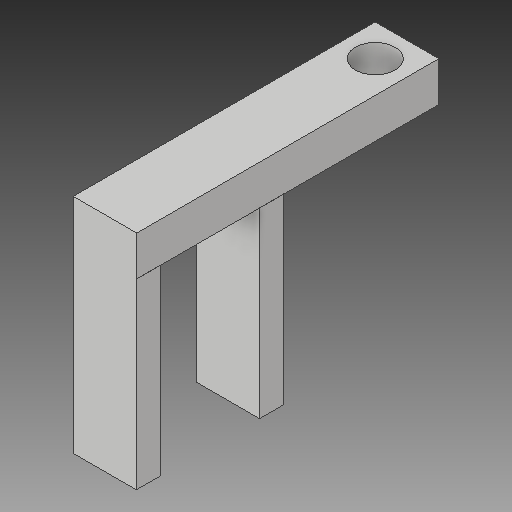
# Autodesk Inventor part: A1
Saved by Autodesk Inventor 2019 (Build 230136000, 136)
## iProperties
Created: 2020-03-28
Part Number: A1
Material: Generic
Document SubType Name: Modeling
Designer: Pulag
Density: 1 g/cm^3
Appearance: Default
Author: Pulag
Autodesk Inventor part; units mm, degrees
ref_plane "YZ Plane" through (0, 0, 0) normal (1, 0, 0) x (0, 1, 0)
ref_plane "XZ Plane" through (0, 0, 0) normal (0, 1, 0) x (-1, 0, 0)
ref_plane "XY Plane" through (0, 0, 0) normal (0, 0, 1) x (1, 0, 0)
sketch "Sketch1" plane through (0, 0, 0) normal (0, 1, 0) x (-1, 0, 0)
  point P0 (0, 0)
sketch "Sketch2" plane through (-2.6971, 0, -13.0721) normal (0, 1, 0) x (-1, 0, 0)
  circle A0 centre (-1.6971, 1.6971) radius 2.5
  line L0 (2.3029, 5.6971) -> (-5.6971, 5.6971)
  line L1 (-5.6971, 5.6971) -> (-5.6971, -2.3029)
  line L2 (-5.6971, -2.3029) -> (2.3029, -2.3029)
  line L3 (2.3029, -2.3029) -> (2.3029, 5.6971)
  line L4 (2.3029, 5.6971) -> (-5.6971, -2.3029) construction
  line L5 (-5.6971, 5.6971) -> (2.3029, -2.3029) construction
  line L6 (2.3029, 5.6971) -> (-5.6971, 5.6971)
  line L7 (-5.6971, 5.6971) -> (-5.6971, 35.6971)
  line L8 (-5.6971, 35.6971) -> (2.3029, 35.6971)
  line L9 (2.3029, 35.6971) -> (2.3029, 5.6971)
  point P0 (-7.6971, -4.5529)
  dimension "d3" = 5
  dimension "d1" = 8
  dimension "d2" = 8
  dimension "d0" = 30
  constraints: 20 end point, 4 parallel, 2 horizontal, 2 midpoint, 2 perpendicular, 1 centre point, 1 coincident
  measures "d3" diameter of A0
  measures "d1" distance of L2.end L1.end
  measures "d2" distance of L1.end L0.end
  measures "d0" distance of L6.end L7.end
extrude "Extrusion1" add sketch "Sketch2" along normal blind 5
sketch "Sketch3" plane through (-2.6971, 0, -13.0721) normal (0, -1, 0) x (1, 0, 0)
  line L0 (-2.3029, -2.3029) -> (-2.3029, 35.6971) projected
  line L1 (5.6449, 20.1971) -> (-2.3029, 20.1971)
  line L2 (-2.3029, 20.1971) -> (-2.3029, 17.1971)
  line L3 (-2.3029, 17.1971) -> (5.6449, 17.1971)
  line L4 (5.6449, 17.1971) -> (5.6449, 20.1971)
  line L5 (5.6449, 32.6971) -> (-2.3029, 32.6971)
  line L6 (-2.3029, 32.6971) -> (-2.3029, 35.6971)
  line L7 (-2.3029, 35.6971) -> (5.6449, 35.6971)
  line L8 (5.6449, 35.6971) -> (5.6449, 32.6971)
  point P0 (2.6971, 13.0721)
  dimension "d7" = 3
  dimension "d11" = 12.5
  dimension "d12" = 3
  constraints: 16 end point, 4 parallel, 2 horizontal, 2 perpendicular, 2 point on line
  measures "d7" distance of L2.end L1.end
  measures "d11" distance between parallel lines of L5 L1
  measures "d12" distance between parallel lines of L7 L5
extrude "Extrusion2" add sketch "Sketch3" along normal blind 23
sketch "Sketch4" plane through (-5, 0, -15.375) normal (-1, 0, 0) x (0, 0, 1)
  point P0 (15.375, 0)
body "Solid1"
